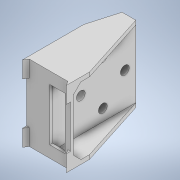
# Autodesk Inventor part: finger_v1
Saved by Autodesk Inventor 2022 (Build 260153000, 153)
## iProperties
Created: 2022-06-04
Part Number: finger_v1
Material: Generic
Document SubType Name: Modeling
Designer: kylem
Density: 1 g/cm^3
Appearance: Default
Author: kylem
Autodesk Inventor part; units mm, degrees
ref_plane "YZ Plane" through (0, 0, 0) normal (1, 0, 0) x (0, 1, 0)
ref_plane "XZ Plane" through (0, 0, 0) normal (0, 1, 0) x (-1, 0, 0)
ref_plane "XY Plane" through (0, 0, 0) normal (0, 0, 1) x (1, 0, 0)
sketch "Sketch1" plane through (0, 0, 0) normal (0, 1, 0) x (-1, 0, 0)
  line L0 (0, 0) -> (0, -30.6)
  line L1 (0, -30.6) -> (5, -30.6)
  line L2 (0, 0) -> (13.774, 0)
  line L3 (13.774, 0) -> (5, -30.6)
  line L4 (13.774, 0) -> (13.774, 4)
  line L5 (0, 0) -> (0, 9.5471)
  line L6 (13.774, 4) -> (-10.8744, 4)
  point P0 (0, 4)
  dimension "d0" = 30.6
  dimension "d1" = 5
  dimension "d2" = 13.774
  dimension "d3" = 4
  constraints: 14 end point, 2 horizontal, 2 perpendicular, 2 vertical
  measures "d0" distance of L0.start L0.end
  measures "d1" distance of L0.end L1.end
  measures "d2" distance of L0.start L2.end
  measures "d3" distance of L2.end L4.end
extrude "Extrusion1" add sketch "Sketch1" along normal blind 24
sketch "Sketch2" plane through (0, 0, 4) normal (1, 0, 0) x (0, 0, -1)
  line L0 (34.6, 0) -> (34.6, 24) projected
  line L1 (34.6, 12) -> (30.6, 12)
  line L2 (30.6, 12) -> (14.6, 12)
  line L3 (22.6, 12) -> (22.6, 20)
  line L4 (22.6, 12) -> (22.6, 4)
  circle A0 centre (22.6, 20) radius 1.6
  circle A1 centre (14.6, 12) radius 1.6
  circle A2 centre (22.6, 4) radius 1.6
  circle A3 centre (30.6, 12) radius 1.6
  point P0 (4, 0)
  dimension "d6" = 4
  dimension "d7" = 16
  dimension "d8" = 8
  dimension "d9" = 8
  dimension "d10" = 3.2
  dimension "d11" = 3.2
  dimension "d12" = 3.2
  dimension "d13" = 3.2
  constraints: 8 end point, 4 centre point, 4 coincident, 2 horizontal, 2 midpoint, 2 vertical
  measures "d6" distance of L1.start L1.end
  measures "d7" distance of L1.end L2.end
  measures "d8" distance of L3.start L3.end
  measures "d9" distance of L3.start L4.end
  measures "d10" diameter of A0
  measures "d11" diameter of A1
  measures "d12" diameter of A2
  measures "d13" diameter of A3
extrude "Extrusion2" cut sketch "Sketch2" against normal blind 24
ref_plane "Work Plane1" through (-3, 0, 4) normal (1, 0, 0) x (0, 0, -1)
sketch "Sketch3" plane through (-3, 0, 4) normal (1, 0, 0) x (0, 0, -1)
  circle A0 centre (22.6, 20) radius 1.6 projected
  circle A1 centre (22.6, 20) radius 2.95
  circle A2 centre (14.6, 12) radius 1.6 projected
  circle A3 centre (14.6, 12) radius 2.95
  circle A4 centre (22.6, 4) radius 1.6 projected
  circle A5 centre (22.6, 4) radius 2.95
  circle A6 centre (30.6, 12) radius 1.6 projected
  circle A7 centre (30.6, 12) radius 2.95
  point P0 (4, 0)
  dimension "d17" = 5.9
  dimension "d18" = 5.9
  dimension "d19" = 5.9
  dimension "d20" = 5.9
  constraints: 4 centre point, 4 coincident
  measures "d17" diameter of A1
  measures "d18" diameter of A3
  measures "d19" diameter of A5
  measures "d20" diameter of A7
extrude "Extrusion3" cut sketch "Sketch3" against normal blind 24 contours A0 | A1 | A2 | A3 | A4 | A5 | A6 | A7
sketch "Sketch5" plane through (0, 0, 4) normal (1, 0, 0) x (0, 0, -1)
  line L0 (4, 0) -> (0, 0) projected
  line L1 (34.6, 24) -> (4, 24) projected
  line L2 (0, 0) -> (4, 0)
  line L3 (4, 0) -> (4, 24)
  line L4 (4, 24) -> (0, 24)
  line L5 (0, 24) -> (0, 0)
  line L6 (4, 0) -> (4, 24) projected
  line L7 (4, 24) -> (6.5, 24)
  line L8 (6.5, 24) -> (6.5, 21.5)
  line L9 (6.5, 21.5) -> (4, 21.5)
  line L10 (4, 21.5) -> (4, 24)
  line L11 (4, 0) -> (6.5, 0)
  line L12 (6.5, 0) -> (6.5, 2.5)
  line L13 (6.5, 2.5) -> (4, 2.5)
  line L14 (4, 2.5) -> (4, 0)
  line L15 (4, 2.5) -> (6.5, 0)
  line L16 (4, 21.5) -> (6.5, 24)
  dimension "d40" = 4
  dimension "d41" = 24
  dimension "d44" = 2.5
  dimension "d45" = 2.5
  dimension "d46" = 2.5
  dimension "d47" = 2.5
  constraints: 28 end point, 6 parallel, 3 horizontal, 3 perpendicular
  measures "d40" distance of L4.end L1.end
  measures "d41" distance of L1.end L2.end
  measures "d44" distance of L8.end L9.end
  measures "d45" distance of L7.end L8.end
  measures "d46" distance of L13.end L12.end
  measures "d47" distance of L12.end L11.end
extrude "Extrusion6" add sketch "Sketch5" along normal blind 8.9 contours L0 L5 L4 L3 | L3 L15 L11 | L3 L1 L16
sketch "Sketch7" plane through (0, 2.5, 0) normal (0, 0, -1) x (-1, 0, 0)
  line L0 (0, 0) -> (-8.9, 0) projected
  line L1 (0, 19) -> (-8.9, 19) projected
  line L2 (0, 0) -> (-5.5, 0)
  line L3 (-5.5, 0) -> (-5.5, 19)
  line L4 (-5.5, 19) -> (0, 19)
  line L5 (0, 19) -> (0, 0)
  line L6 (0, 21.5) -> (0, 19) projected
  line L7 (0, 19) -> (-0.3, 19)
  line L8 (-0.3, 19) -> (-0.3, 0)
  line L9 (-0.3, 0) -> (0, 0)
  line L10 (0, 0) -> (0, 19)
  point P0 (0, -2.5)
  dimension "d55" = 5.5
  dimension "d56" = 0.3
  constraints: 16 end point, 4 parallel, 2 horizontal, 2 perpendicular, 2 point on line
  measures "d55" distance of L3.end L4.end
  measures "d56" distance of L9.end L8.end
extrude "Extrusion8" cut sketch "Sketch7" against normal blind 30 contours L0 L3 L1 L8
sketch "Sketch9" plane through (-13.774, 0, 0) normal (-1, 0, 0) x (0, 0, 1)
  line L0 (-2.5, 24) -> (-30.6, 24) projected
  line L1 (4, 0) -> (-30.6, 0)
  line L2 (-30.6, 0) -> (-30.6, 24)
  line L3 (-30.6, 24) -> (4, 24)
  line L4 (4, 24) -> (4, 0)
  point P0 (0, 0)
  constraints: 8 end point, 2 parallel, 1 horizontal, 1 perpendicular
extrude "Extrusion10" cut sketch "Sketch9" against normal blind 5.674
sketch "Sketch10" plane through (8.9, 0, 4) normal (1, 0, 0) x (0, 0, -1)
  line L0 (6.5, 24) -> (0, 24) projected
  line L1 (0, 24) -> (0, 24.25)
  line L2 (0, 24.25) -> (8.0681, 24.25)
  line L3 (4, 21.5) -> (6.5, 24) projected
  line L4 (4, 21.5) -> (7.5355, 25.0355)
  line L5 (4, 21.5) -> (9, 21.5) construction
  line L6 (0, 24) -> (0, 0) projected
  line L7 (6.5, 24) -> (0, 24)
  line L8 (4, 21.5) -> (4, 2.5) projected
  line L9 (4, 12) -> (-3.3365, 12)
  line L10 (6.5, 0) -> (0, 0)
  line L11 (0, 0) -> (0, -0.25)
  line L12 (0, -0.25) -> (8.0681, -0.25)
  line L13 (4, 2.5) -> (6.5, 0)
  line L14 (4, 2.5) -> (7.5355, -1.0355)
  line L15 (4, 2.5) -> (9, 2.5) construction
  line L16 (6.5, 0) -> (0, 0)
  point P0 (4, 0)
  point P1 (6.75, -0.25)
  point P2 (6.75, 24.25)
  dimension "d65" = 0.25
  dimension "d66" = 5
  dimension "d67" = 45
  constraints: 26 end point, 5 symmetric about line, 2 horizontal, 2 perpendicular, 1 equal length, 1 midpoint, 1 vertical
  measures "d65" distance of L0.end L1.end
  measures "d66" distance of L3.start L4.end
  measures "d67" angle of L5 L4
extrude "Extrusion11" add sketch "Sketch10" against normal blind 8.9 contours L0 L1 L2 L4 | L10 L14 L12 L11
ref_plane "Work Plane2" through (0, 12, 0) normal (0, -1, 0) x (1, 0, 0)
sketch "Sketch12" plane through (8.9, -0.25, -2.75) normal (0, -1, 0) x (1, 0, 0)
  line L0 (0, 0) -> (0, 2.75) projected
  line L1 (0, 0) -> (-8.9, 0)
  line L2 (-8.9, 0) -> (-8.9, 6.75)
  line L3 (-8.9, 6.75) -> (0, 6.75)
  line L4 (0, 6.75) -> (0, 0)
  point P0 (-8.9, 2.75)
  constraints: 8 end point, 2 parallel, 1 horizontal, 1 perpendicular
extrude "Extrusion12" add sketch "Sketch12" along normal blind 1.5
sketch "Sketch13" plane through (0, 0, 0) normal (0, -1, 0) x (1, 0, 0)
  line L0 (0, -30.6) -> (-5, -30.6) projected
  line L1 (0, -2.5) -> (0, 4) projected
  line L2 (-5, -30.6) -> (0, -30.6)
  line L3 (0, -30.6) -> (0, 4)
  line L4 (0, 4) -> (-5, 4)
  line L5 (-5, 4) -> (-5, -30.6)
  line L6 (-8.1, -19.7885) -> (-5, -19.7885)
  line L7 (-5, -19.7885) -> (-5, 4)
  line L8 (-5, 4) -> (-8.1, 4)
  line L9 (-8.1, 4) -> (-8.1, -19.7885)
  line L10 (-5, -30.6) -> (-8.1, -19.7885) projected
  line L11 (-5, -30.6) -> (-8.1, -19.7885)
  point P0 (0, 0)
  constraints: 18 end point, 5 equal length, 2 horizontal, 2 perpendicular
extrude "Extrusion13" add sketch "Sketch13" along normal blind 1.75
sketch "Sketch14" plane through (8.9, -1.75, -2.75) normal (0, -1, 0) x (1, 0, 0)
  line L0 (-8.9, -27.85) -> (-8.9, 0) projected
  line L1 (0, 0) -> (0, 2.75) projected
  line L2 (-8.9, -27.85) -> (0, 0)
  line L3 (-8.9, -27.85) -> (0, -27.85)
  line L4 (0, -27.85) -> (0, 0)
  line L5 (0, 0) -> (-8.9, 0)
  line L6 (-8.9, 0) -> (-8.9, -27.85)
  point P0 (-8.9, 2.75)
  point P1 (-8.9, 0)
  constraints: 10 end point, 2 parallel, 1 horizontal, 1 perpendicular
extrude "Extrusion14" add sketch "Sketch14" against normal blind 1.5 contours L0 L5 L2
mirror "Mirror1" about plane through (0, 12, 0) normal (0, -1, 0) of "Extrusion12", "Extrusion13", "Extrusion14"
sketch "Sketch15" plane through (8.9, 0, 4) normal (1, 0, 0) x (0, 0, -1)
  line L0 (22.1903, 31.1847) -> (-2.991, 31.1847)
  line L1 (-2.991, 31.1847) -> (-2.991, -5.1617)
  line L2 (-2.991, -5.1617) -> (22.1903, -5.1617)
  line L3 (22.1903, -5.1617) -> (22.1903, 31.1847)
  point P0 (4, 0)
  constraints: 8 end point, 2 parallel, 1 horizontal, 1 perpendicular
extrude "Extrusion17" cut sketch "Sketch15" against normal blind 1
sketch "Sketch16" plane through (-8.1, -1.75, 4) normal (0, 0, 1) x (1, 0, 0)
  line L0 (23.1984, -4.3461) -> (-2.2485, -4.3461)
  line L1 (-2.2485, -4.3461) -> (-2.2485, 32.2961)
  line L2 (-2.2485, 32.2961) -> (23.1984, 32.2961)
  line L3 (23.1984, 32.2961) -> (23.1984, -4.3461)
  point P0 (8.1, 1.75)
  constraints: 8 end point, 2 parallel, 1 horizontal, 1 perpendicular
extrude "Extrusion18" cut sketch "Sketch16" against normal blind 3
sketch "Sketch17" plane through (5.5, 2.5, 0) normal (0, 0, -1) x (-1, 0, 0)
  line L0 (5.2, 0) -> (0, 0) projected
  line L1 (-2.4, 19) -> (-2.4, 0) projected
  line L2 (0, 0) -> (-2.4, 0)
  line L3 (-2.4, 0) -> (-2.4, 19)
  line L4 (-2.4, 19) -> (0, 19)
  line L5 (0, 19) -> (0, 0)
  point P0 (5.5, -2.5)
  constraints: 8 end point, 2 parallel, 1 horizontal, 1 perpendicular
extrude "Extrusion19" cut sketch "Sketch17" against normal blind 3
sketch "Sketch18" plane through (8.9, -1.75, -2.75) normal (0, -1, 0) x (1, 0, 0)
  line L0 (-8.6, 3.75) -> (-1, 3.75) projected
  line L1 (-1, 3.75) -> (-3, 3.75)
  line L2 (-1, 5.75) -> (-1, 3.75)
  line L3 (-1, 3.75) -> (-2, 3.75)
  line L4 (-2, 3.75) -> (-2, 5.25)
  line L5 (-2, 5.25) -> (-1, 5.25)
  line L6 (-1, 5.25) -> (-1, 3.75)
  line L7 (-1, 5.25) -> (-2, 3.75)
  point P0 (-8.9, 2.75)
  point P1 (-2, 3.75)
  dimension "d97" = 1
  dimension "d98" = 1.5
  constraints: 14 end point, 2 horizontal, 2 parallel, 1 perpendicular
  measures "d97" distance of L4.end L5.end
  measures "d98" distance of L3.end L4.end
extrude "Extrusion20" add sketch "Sketch18" against normal blind 27.5 contours L7 L2 L0
sketch "Sketch19" plane through (7.9, 2.5, 1) normal (0, 0, -1) x (-1, 0, 0)
  line L0 (7.6, 19) -> (0, 19) projected
  line L1 (7.6, 0) -> (0, 0) projected
  line L2 (0, 19) -> (2, 19)
  line L3 (2, 19) -> (2, 0)
  line L4 (2, 0) -> (0, 0)
  line L5 (0, 0) -> (0, 19)
  point P0 (7.9, -2.5)
  dimension "d101" = 2
  constraints: 8 end point, 2 parallel, 1 horizontal, 1 perpendicular, 1 point on line
  measures "d101" distance of L3.end L4.end
extrude "Extrusion21" add sketch "Sketch19" along normal blind 1
sketch "Sketch20" plane through (8.9, -1.75, -2.75) normal (0, -1, 0) x (1, 0, 0)
  line L0 (-1, 5.25) -> (-1, -3.1292) projected
  line L1 (-1, 5.25) -> (-17, 5.25)
  line L2 (-17, 5.25) -> (-17, 0.25)
  line L3 (-17, 5.25) -> (-16, 5.25)
  line L4 (-16, 5.25) -> (-16, 3.75)
  line L5 (-16, 3.75) -> (-17, 3.75)
  line L6 (-17, 3.75) -> (-17, 5.25)
  line L7 (-17, 5.25) -> (-16, 3.75)
  point P0 (-8.9, 2.75)
  dimension "d107" = 16
  dimension "d108" = 5
  dimension "d109" = 1
  dimension "d110" = 1.5
  constraints: 14 end point, 2 horizontal, 2 parallel, 2 perpendicular
  measures "d107" distance of L0.start L1.end
  measures "d108" distance of L1.end L2.end
  measures "d109" distance of L4.end L5.end
  measures "d110" distance of L3.end L4.end
extrude "Extrusion22" add sketch "Sketch20" against normal blind 27.5 contours L7 L5 L2
sketch "Sketch21" plane through (7.9, 0, 4) normal (1, 0, 0) x (0, 0, -1)
  line L0 (1.5, -1.75) -> (1.5, 25.75) projected
  line L1 (1.5, -1.75) -> (1.5, 4.25)
  line L2 (1.5, 25.75) -> (9.8792, 25.75) projected
  line L3 (1.5, 25.75) -> (1.5, 19.75)
  line L4 (1.5, 19.75) -> (3, 19.75)
  line L5 (3, 21.5) -> (3, 2.5) projected
  line L6 (1.5, 19.75) -> (1.5, 4.25)
  line L7 (1.5, 4.25) -> (3, 4.25)
  line L8 (3, 4.25) -> (3, 19.75)
  point P0 (4, 0)
  dimension "d116" = 6
  dimension "d117" = 6
  constraints: 12 end point, 3 point on line, 2 perpendicular, 1 collinear, 1 horizontal
  measures "d116" distance of L0.start L1.end
  measures "d117" distance of L0.end L3.end
extrude "Extrusion23" cut sketch "Sketch21" against normal blind 60
body "Solid1"
